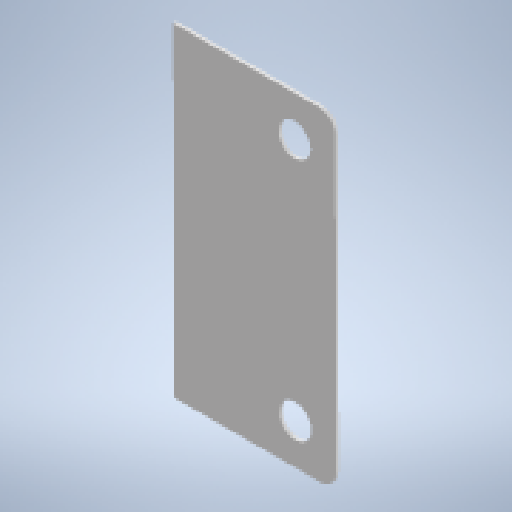
# Autodesk Inventor part: Top Stiffener
Saved by Autodesk Inventor 2025 (Build 290162000, 162)
## iProperties
Created: 2024-11-12
Part Number: Top Stiffener
Material: Generic
Document SubType Name: Modeling
Designer: Caleb Fangmeier
Density: 1 g/cm^3
Appearance: Default
Author: Caleb Fangmeier
Autodesk Inventor part; units mm, degrees
ref_plane "YZ Plane" through (0, 0, 0) normal (1, 0, 0) x (0, 1, 0)
ref_plane "XZ Plane" through (0, 0, 0) normal (0, 1, 0) x (-1, 0, 0)
ref_plane "XY Plane" through (0, 0, 0) normal (0, 0, 1) x (1, 0, 0)
sketch "Sketch1" plane through (0, 0, 0) normal (0, 0, 1) x (1, 0, 0)
  line L0 (-92.084, -158.9648) -> (-92.1426, -140.9593)
  line L1 (-93.1425, -139.9627) -> (-119.7195, -139.9627)
  arc A0 (-92.1426, -140.9593) -> (-93.1425, -139.9628) centre (-93.1424, -140.9626) ccw
  arc A1 (-93.084, -159.9622) -> (-92.084, -158.9648) centre (-93.084, -158.9622) ccw
  circle A2 centre (-94.589, -157.4672) radius 1
  circle A3 centre (-94.6377, -142.4676) radius 1
  line L2 (-133.7975, -159.9622) -> (-93.084, -159.9622)
  line L3 (-102.1459, -139.9627) -> (-102.0808, -159.9622)
  line L4 (-102.0808, -159.9622) -> (-93.084, -159.9622)
  line L5 (-102.1459, -139.9627) -> (-93.1425, -139.9628)
  arc A4 (-92.1426, -140.9593) -> (-93.1425, -139.9628) centre (-93.1424, -140.9626) ccw
  arc A5 (-93.084, -159.9622) -> (-92.084, -158.9648) centre (-93.084, -158.9622) ccw
  line L6 (-92.084, -158.9648) -> (-92.1426, -140.9593)
  point P0 (0, 0)
extrude "Extrusion1" add sketch "Sketch1" along normal blind 0.2
body "Solid1"
